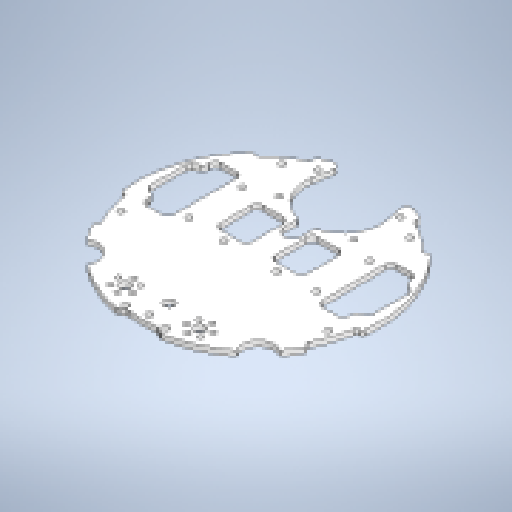
# Autodesk Inventor part: Top Plate
Saved by Autodesk Inventor 2023.2 (Build 272271000, 271)
## iProperties
Created: 2022-12-28
Part Number: Top Plate
Material: UHMW, White
Document SubType Name: Modeling
Designer: Nathan Cai
Mass: 29.6891 g
Surface Area: 260.075 cm^2
Volume: 31.5842 cm^3
Density: 0.94 g/cm^3
Appearance: Smooth - White
Author: Nathan Cai
Autodesk Inventor part; units mm, degrees
ref_plane "YZ Plane" through (0, 0, 0) normal (1, 0, 0) x (0, 1, 0)
ref_plane "XZ Plane" through (0, 0, 0) normal (0, 1, 0) x (-1, 0, 0)
ref_plane "XY Plane" through (0, 0, 0) normal (0, 0, 1) x (1, 0, 0)
sketch "Sketch1" plane through (0, 0, 0) normal (0, 1, 0) x (-1, 0, 0)
  circle A0 centre (0, 0) radius 73.025
  line L0 (0, 0) -> (0, -73.025) construction
  line L1 (0, 0) -> (-12.6807, -71.9156)
  line L2 (0, 0) -> (12.6807, -71.9156)
  line L3 (0, 0) -> (52.5298, -50.7274)
  line L4 (0, 0) -> (32.0121, -65.6344)
  line L5 (0, 0) -> (72.3143, -10.1631)
  line L6 (0, 0) -> (64.4772, -34.2832)
  line L7 (0, 0) -> (64.4772, 34.2832)
  line L8 (0, 0) -> (72.3143, 10.1631)
  line L9 (0, 0) -> (32.0121, 65.6344)
  line L10 (0, 0) -> (52.5298, 50.7274)
  circle A1 centre (0, 0) radius 69.85
  line L11 (0, 0) -> (-12.6807, 71.9156)
  line L12 (0, 0) -> (12.6807, 71.9156)
  line L13 (0, 0) -> (-52.5298, 50.7274)
  line L14 (0, 0) -> (-32.0121, 65.6344)
  line L15 (0, 0) -> (-72.3143, 10.1631)
  line L16 (0, 0) -> (-64.4772, 34.2832)
  line L17 (0, 0) -> (-64.4772, -34.2832)
  line L18 (0, 0) -> (-72.3143, -10.1631)
  line L19 (0, 0) -> (-32.0121, -65.6344)
  line L20 (0, 0) -> (-52.5298, -50.7274)
  point P0 (30.6202, -62.7808)
  point P1 (50.2459, -48.5219)
  point P2 (52.5298, -50.7274)
  point P3 (64.4772, -34.2832)
  point P4 (61.6739, -32.7926)
  point P5 (69.1702, -9.7212)
  point P6 (72.3143, -10.1631)
  point P7 (72.3143, 10.1631)
  point P8 (69.1702, 9.7212)
  point P9 (61.6739, 32.7926)
  point P10 (52.5298, 50.7274)
  point P11 (50.2459, 48.5219)
  point P12 (30.6202, 62.7808)
  point P13 (-12.1293, -68.7888)
  point P14 (12.1293, -68.7888)
  point P15 (12.6807, -71.9156)
  point P16 (32.0121, -65.6344)
  point P17 (12.1293, 68.7888)
  point P18 (-12.1293, 68.7888)
  point P19 (-12.6807, 71.9156)
  point P20 (-64.4772, 34.2832)
  point P21 (-61.6739, 32.7926)
  point P22 (-69.1702, 9.7212)
  point P23 (-52.5298, -50.7274)
  point P24 (-50.2459, -48.5219)
  point P25 (-30.6202, -62.7808)
  dimension "d0" = 146.05
  dimension "d1" = 10
  dimension "d4" = 360
  dimension "d160" = 139.7
  constraints: 42 end point, 4 coincident, 2 centre point, 2 point on circle, 1 symmetric about line, 1 vertical, 49 other
  measures "d0" diameter of A0
  measures "d1" angle of L0 L1
  measures "d160" diameter of A1
extrude "Extrusion1" add sketch "Sketch1" along normal blind 3.175 contours A0 L5 A1 L8 | A0 L6 A1 L5 | L7 A1 L10 A0 | A1 L5 L8 | L8 L7 A1 | A0 L3 A1 L6 | A1 L6 L5 | L10 A1 L9 A0 | L7 L10 A1 | L2 A1 L1 | L4 A1 L2 | L6 A1 L3 | L3 A1 L4 | L12 A1 L9 | L9 A1 L10 | L14 A1 L11 | L11 A1 L12 | L16 A1 L13 | L13 A1 L14 | L18 A1 L15 | L15 A1 L16 | L20 A1 L17 | L17 A1 L18 | L1 A1 L19 | L19 A1 L20 | L9 A1 L12 A0 | A1 L2 A0 L1 | L1 A0 L19 A1 | A1 L4 A0 L2 | A1 L14 A0 L11 | L13 A0 L14 A1 | A1 L16 A0 L13 | A1 L18 A0 L15 | L17 A0 L18 A1 | A1 L20 A0 L17
sketch "Sketch4" plane through (0, 3.175, 0) normal (0, 1, 0) x (1, 0, 0)
  line L0 (0, 0) -> (0, 66.675) construction
  line L1 (-44.45, 26.9875) -> (44.45, 26.9875) construction
  line L2 (44.45, 26.9875) -> (44.45, -1.5875)
  line L3 (44.45, -1.5875) -> (-44.45, -1.5875) construction
  line L4 (-44.45, -1.5875) -> (-44.45, 26.9875)
  line L5 (-44.45, 26.9875) -> (44.45, -1.5875) construction
  line L6 (44.45, 26.9875) -> (-44.45, -1.5875) construction
  line L7 (-44.45, 12.7) -> (44.45, 12.7) construction
  line L8 (-66.675, 34.925) -> (-44.45, 34.925)
  line L9 (-44.45, 34.925) -> (-44.45, -9.525)
  line L10 (-44.45, -9.525) -> (-66.675, -9.525)
  line L11 (-66.675, -9.525) -> (-66.675, 34.925)
  line L12 (-66.675, 34.925) -> (-44.45, -9.525) construction
  line L13 (-44.45, 34.925) -> (-66.675, -9.525) construction
  line L14 (44.45, -1.5875) -> (44.45, 26.9875)
  line L15 (66.675, 34.925) -> (44.45, 34.925)
  line L16 (44.45, 34.925) -> (44.45, -9.525)
  line L17 (44.45, -9.525) -> (66.675, -9.525)
  line L18 (66.675, -9.525) -> (66.675, 34.925)
  line L19 (66.675, 34.925) -> (44.45, -9.525) construction
  line L20 (44.45, 34.925) -> (66.675, -9.525) construction
  line L21 (38.1, 12.7) -> (38.1, 28.575) construction
  circle A0 centre (38.1, 28.575) radius 1.7526
  circle A1 centre (38.1, -3.175) radius 1.7526
  circle A2 centre (-38.1, 28.575) radius 1.7526
  circle A3 centre (-38.1, -3.175) radius 1.7526
  line L22 (-66.675, 34.925) -> (-60.325, 34.925)
  line L23 (-60.325, 34.925) -> (-60.325, 28.575)
  line L24 (-60.325, 28.575) -> (-66.675, 28.575) construction
  line L25 (-66.675, 28.575) -> (-66.675, 34.925)
  line L26 (-60.325, 28.575) -> (-66.675, 24.9088)
  line L27 (-60.325, -9.525) -> (-60.325, -3.175)
  line L28 (-60.325, -3.175) -> (-66.675, 0.4912)
  line L29 (60.325, 34.925) -> (60.325, 28.575)
  line L30 (60.325, 28.575) -> (66.675, 24.9088)
  line L31 (60.325, -9.525) -> (60.325, -3.175)
  line L32 (60.325, -3.175) -> (66.675, 0.4912)
  line L33 (-38.1, -3.175) -> (38.1, -3.175) construction
  circle A4 centre (-15.875, -4.7625) radius 1.7526
  circle A5 centre (15.875, -4.7625) radius 1.7526
  line L34 (-26.0625, 25.4) -> (-7.0125, 25.4)
  line L35 (-7.0125, 25.4) -> (-7.0125, 0)
  line L36 (-7.0125, 0) -> (-26.0625, 0)
  line L37 (-26.0625, 0) -> (-26.0625, 25.4)
  line L38 (-26.0625, 25.4) -> (-7.0125, 0) construction
  line L39 (-7.0125, 25.4) -> (-26.0625, 0) construction
  line L40 (26.0625, 25.4) -> (7.0125, 25.4)
  line L41 (7.0125, 25.4) -> (7.0125, 0)
  line L42 (7.0125, 0) -> (26.0625, 0)
  line L43 (26.0625, 0) -> (26.0625, 25.4)
  line L44 (26.0625, 25.4) -> (7.0125, 0) construction
  line L45 (7.0125, 25.4) -> (26.0625, 0) construction
  circle A6 centre (22.225, -57.15) radius 3.175
  line L46 (22.225, -57.15) -> (28.2642, -55.1877) construction
  circle A7 centre (28.2642, -55.1877) radius 1.5875
  line L47 (22.225, -57.15) -> (22.225, -53.975) construction
  circle A8 centre (26.944, -61.399) radius 1.5875
  circle A9 centre (20.9048, -63.3612) radius 1.5875
  circle A10 centre (16.1858, -59.1123) radius 1.5875
  circle A11 centre (17.506, -52.901) radius 1.5875
  circle A12 centre (23.5452, -50.9388) radius 1.5875
  circle A13 centre (-22.225, -57.15) radius 3.175
  line L48 (-22.225, -57.15) -> (-28.2642, -55.1877) construction
  circle A14 centre (-28.2642, -55.1877) radius 1.5875
  line L49 (-22.225, -57.15) -> (-22.225, -53.975) construction
  circle A15 centre (-26.944, -61.399) radius 1.5875
  circle A16 centre (-20.9048, -63.3612) radius 1.5875
  circle A17 centre (-16.1858, -59.1123) radius 1.5875
  circle A18 centre (-17.506, -52.901) radius 1.5875
  circle A19 centre (-23.5452, -50.9388) radius 1.5875
  point P0 (0, 12.7)
  point P1 (-55.5625, 12.7)
  point P2 (55.5625, 12.7)
  point P3 (44.45, -1.5875)
  point P4 (0, 12.7)
  point P5 (-66.675, 0.4912)
  point P6 (-60.325, -9.525)
  point P7 (-60.325, 34.925)
  point P8 (60.325, -9.525)
  point P9 (66.675, 0.4912)
  point P10 (60.325, 34.925)
  point P11 (-16.5375, 12.7)
  point P12 (16.5375, 12.7)
  dimension "d108" = 6.35
  dimension "d30" = 88.9
  dimension "d31" = 28.575
  dimension "d34" = 22.225
  dimension "d35" = 44.45
  dimension "d52" = 6.35
  dimension "d53" = 15.875
  dimension "d54" = 3.5052
  dimension "d63" = 12.7
  dimension "d64" = 6.35
  dimension "d65" = 6.35
  dimension "d66" = 30
  dimension "d78" = 3.5052
  dimension "d79" = 15.875
  dimension "d80" = 17.4625
  dimension "d104" = 19.05
  dimension "d105" = 25.4
  dimension "d107" = 18.3875
  dimension "d109" = 22.225
  dimension "d110" = 69.85
  dimension "d111" = 6.35
  dimension "d112" = 3.175
  dimension "d113" = 72
  dimension "d116" = 360
  constraints: 100 end point, 32 symmetric about line, 18 centre point, 11 midpoint, 8 parallel, 5 horizontal, 5 point on line, 4 perpendicular, 4 vertical, 3 coincident, 2 vertical alignment, 27 other
  measures "d30" distance of L2.end L3.end
  measures "d31" distance between parallel lines of L3 L1
  measures "d34" distance of L9.end L10.end
  measures "d35" distance of L8.end L9.end
  measures "d52" distance between parallel lines of L16 L21
  measures "d53" distance from line of L7 L21.end
  measures "d54" diameter of A0
  measures "d63" distance of point (0, 12.7) L0.start
  measures "d64" distance of L23.end L24.end
  measures "d65" distance of L22.end L23.end
  measures "d66" angle of L24 L26
  measures "d78" diameter of A4
  measures "d79" distance from line of L0 A4.centre
  measures "d80" distance from line of L7 A4.centre
  measures "d104" distance of L35.end L36.end
  measures "d105" distance of L34.end L35.end
  measures "d107" distance between parallel lines of L4 L37
  measures "d109" horizontal distance of point (0, 12.7) L46.start
  measures "d110" vertical distance of L46.start point (0, 12.7)
  measures "d111" distance of L46.start L46.end
  measures "d112" diameter of A7
  measures "d113" angle of L47 L46
extrude "Extrusion2" cut sketch "Sketch4" against normal through all contours L16 L15 L29 L30 L18 L32 L31 L17 L2 | L9 L10 L27 L28 L11 L26 L23 L8 L4 | A0 | A1 | A2 | A3 | A4 | A5 | L34 L35 L36 L37 | L43 L42 L41 L40 | A6 | A7 | A8 | A9 | A10 | A11 | A12 | A13 | A14 | A15 | A16 | A17 | A18 | A19
fillet "Fillet2" radius 3.175 24 edges at (-44.45, 1.5875, -34.925) (-44.45, 1.5875, 9.525) (44.45, 1.5875, 9.525) (44.45, 1.5875, -34.925) (60.325, 1.5875, -28.575) (66.675, 1.5875, -24.9088) (66.675, 1.5875, -0.4912) (60.325, 1.5875, 3.175) (-60.325, 1.5875, -28.575) (-66.675, 1.5875, -24.9088) (-66.675, 1.5875, -0.4912) (-60.325, 1.5875, 3.175) (60.325, 1.5875, -34.925) (60.325, 1.5875, 9.525) (-60.325, 1.5875, 9.525) (-60.325, 1.5875, -34.925) (-26.0625, 1.5875, -25.4) (-7.0125, 1.5875, -25.4) (-7.0125, 1.5875, 0) (-26.0625, 1.5875, 0) (7.0125, 1.5875, -25.4) (26.0625, 1.5875, -25.4) (26.0625, 1.5875, 0) (7.0125, 1.5875, 0)
sketch "Sketch5" plane through (0, 3.175, 0) normal (0, 1, 0) x (1, 0, 0)
  line L0 (0, 0) -> (0, 66.675) construction
  circle A0 centre (0, 50.8) radius 22.225
  arc A1 (32.0121, 65.6344) -> (-32.0121, 65.6344) centre (0, 0) ccw projected
  circle A2 centre (0, 50.8) radius 17.4625 construction
  circle A3 centre (-24.6063, 60.325) radius 1.7526
  circle A4 centre (-24.6063, 60.325) radius 3.175 construction
  circle A5 centre (-22.225, 34.925) radius 3.175 construction
  circle A6 centre (-22.225, 34.925) radius 1.7526
  circle A7 centre (24.6063, 60.325) radius 1.7526
  circle A8 centre (24.6063, 60.325) radius 3.175 construction
  circle A9 centre (22.225, 34.925) radius 3.175 construction
  circle A10 centre (22.225, 34.925) radius 1.7526
  arc A11 (32.0121, 65.6344) -> (-32.0121, 65.6344) centre (0, 0) ccw projected
  line L1 (-19.05, 70.4964) -> (-21.8767, 54.7195)
  line L2 (19.05, 70.4964) -> (21.8767, 54.7195)
  circle A12 centre (0, 28.575) radius 4.7625
  line L3 (0, 36.5125) -> (0, 20.6375) construction
  line L4 (-4.7625, 36.5125) -> (-4.7625, 20.6375)
  line L5 (4.7625, 20.6375) -> (4.7625, 36.5125)
  arc A13 (4.7625, 36.5125) -> (-4.7625, 36.5125) centre (0, 36.5125) ccw
  arc A14 (-4.7625, 20.6375) -> (4.7625, 20.6375) centre (0, 20.6375) ccw
  point P0 (-30.5456, -66.3296)
  point P1 (12.6807, -71.9156)
  point P2 (64.4772, -34.2832)
  point P3 (-72.5223, -8.5536)
  point P4 (-19.05, 70.4964)
  point P5 (0, 73.025)
  point P6 (21.8767, 54.7195)
  point P7 (19.05, 70.4964)
  point P8 (-4.7351, 29.0853)
  point P9 (4.7351, 29.0853)
  point P10 (0, 15.875)
  point P11 (4.7625, 28.575)
  point P12 (-4.7625, 28.575)
  dimension "d39" = 34.925
  dimension "d40" = 44.45
  dimension "d41" = 3.5052
  dimension "d42" = 6.35
  dimension "d43" = 9.525
  dimension "d44" = 24.6062
  dimension "d45" = 6.35
  dimension "d46" = 3.5052
  dimension "d47" = 15.875
  dimension "d48" = 22.225
  dimension "d74" = 19.05
  dimension "d102" = 9.525
  dimension "d103" = 12.7
  constraints: 14 end point, 13 centre point, 8 point on circle, 7 tangent, 6 symmetric about line, 5 coincident, 3 point on line, 1 midpoint, 1 parallel, 1 vertical, 4 other
  measures "d39" diameter of A2
  measures "d40" diameter of A0
  measures "d41" diameter of A3
  measures "d42" diameter of A4
  measures "d43" vertical distance of A0.centre A3.centre
  measures "d44" horizontal distance of A0.centre A3.centre
  measures "d45" diameter of A5
  measures "d46" diameter of A6
  measures "d47" vertical distance of A0.centre A6.centre
  measures "d48" horizontal distance of A0.centre A6.centre
  measures "d74" distance from line of L0 L1.start
  measures "d102" diameter of A12
  measures "d103" distance of point (0, 15.875) A12.centre
extrude "Extrusion3" cut sketch "Sketch5" against normal blind 25.4 contours A0 L5 A13 L4 | A0 A1 L2 | A0 A12 L4 A13 L5 | A0 L1 A1 | A12 A0 | A0 A12 | L5 A14 L4 A12 | A3 | A6 | A7 | A10
sketch "Sketch6" plane through (0, 0, 0) normal (0, -1, 0) x (1, 0, 0)
  point P0 (11.8537, 67.2254)
  point P1 (-11.8537, 67.2254)
hole "Hole3" at (11.8537, 0, 67.2254) at (-11.8537, 0, 67.2254) direction (0, 1, 0) diameter 3.5052 end through all
sketch "Sketch7" plane through (0, 3.175, 0) normal (0, 1, 0) x (1, 0, 0)
  arc A0 (12.158, -68.9514) -> (11.3889, -68.9153) centre (11.8537, -67.2254) ccw projected
  circle A1 centre (11.8537, -67.2254) radius 3.302
  arc A2 (-11.3889, -68.9153) -> (-12.158, -68.9514) centre (-11.8537, -67.2254) ccw projected
  circle A3 centre (-11.8537, -67.2254) radius 3.302
  circle A4 centre (11.8537, -67.2254) radius 1.7526
  circle A5 centre (-11.8537, -67.2254) radius 1.7526
  point P0 (0, 0)
  point P1 (12.158, -68.9514)
  point P2 (11.3889, -68.9153)
  dimension "d67" = 6.604
  dimension "d68" = 6.604
  constraints: 4 coincident, 3 centre point, 1 concentric, 3 other
  measures "d67" diameter of A1
  measures "d68" diameter of A3
extrude "Extrusion4" add sketch "Sketch7" against normal up to surface (3.175 mm away)
fillet "Fillet4" radius 1.5875 24 edges at (-12.6807, 1.5875, 71.9156) (-12.427, 1.5875, 70.4773) (-9.235, 1.5875, 69.2368) (12.6807, 1.5875, 71.9156) (12.427, 1.5875, 70.4773) (9.235, 1.5875, 69.2368) (69.1702, 1.5875, 9.7212) (72.3143, 1.5875, 10.1631) (64.4772, 1.5875, 34.2832) (61.6739, 1.5875, 32.7926) (30.6202, 1.5875, -62.7808) (32.0121, 1.5875, -65.6344) (52.5298, 1.5875, -50.7274) (50.2459, 1.5875, -48.5219) (-32.0121, 1.5875, -65.6344) (-30.6202, 1.5875, -62.7808) (-52.5298, 1.5875, -50.7274) (-50.2459, 1.5875, -48.5219) (-72.3143, 1.5875, 10.1631) (-69.1702, 1.5875, 9.7212) (-61.6739, 1.5875, 32.7926) (-64.4772, 1.5875, 34.2832) (-4.7351, 1.5875, -29.0853) (4.7351, 1.5875, -29.0853)
fillet "Fillet5" radius 3.175 2 edges at (19.05, 1.5875, -70.4964) (-19.05, 1.5875, -70.4964)
thicken "Thicken1" operation cut thickness 0.25 both sides no extend neighbours no toward (-0.8477101, 0, -0.5304598) faces at (61.904, 2.1167, 38.7368) (63.0601, 1.0583, 33.5296) (63.8199, 1.0583, 34.4266) (13.1942, 1.0583, 71.6582) (62.9587, 1.0583, 33.4709) (12.2225, 1.0583, 70.9396) (66.7871, 2.1167, 20.4576) (9.8443, 2.1167, 69.8457) (70.7248, 1.0583, 9.9397) (69.8129, 1.0583, 10.0825) (8.7126, 2.1167, 69.3268) (70.965, 1.0583, 9.9551) (6.579, 2.1167, 69.5395) (62.1056, 2.1167, -38.4128) (-8.7126, 2.1167, 69.3268) (51.3752, 1.0583, -49.6125) (52.5834, 1.0583, -50.0545) (-9.8443, 1.0583, 69.8457) (50.9955, 1.0583, -49.3411) (-11.7264, 1.0583, 70.5997) (40.0946, 2.1167, -57.1965) (-12.915, 1.0583, 71.5521) (31.3084, 1.0583, -64.1918) (31.1624, 1.0583, -63.2804) (-45.5793, 2.1167, 57.0541) (31.3571, 1.0583, -64.302) (-63.06, 1.0583, 33.5296) (-63.6672, 1.0583, 34.1) (24.8679, 2.1167, -68.6603) (-62.2411, 1.0583, 31.857) (-63.4147, 2.1167, 29.2848) (-70.7249, 1.0583, 9.9397) (-70.2583, 1.0583, 9.9434) (-72.3414, 1.0583, 9.1242) (-72.823, 2.1167, -5.4282) (-51.3752, 1.0583, -49.6124) (-51.8764, 1.0583, -49.9396) (-49.8575, 1.0583, -49.222) (-42.0072, 2.1167, -55.807) (-31.3084, 1.0583, -64.1918) (-31.8083, 1.0583, -62.207) (-31.1844, 1.0583, -65.7948) (-29.847, 2.1167, -66.6469) (19.9211, 2.1167, -65.8489) (21.2411, 2.1167, -58.2668) (13.984, 1.0583, -33.5258) (5.1613, 1.0583, -28.9021) (4.7625, 1.0583, -23.0416) (-2.0416, 1.0583, -16.3348) (-4.7625, 2.1167, -25.4457) (-5.0189, 2.1167, -28.7148) (-19.7168, 1.0583, -40.5434) (-20.6056, 2.1167, -61.8142) (-19.9361, 2.1167, -65.6043)
sketch "Sketch11" plane through (0, 3.175, 0) normal (0, 1, 0) x (1, 0, 0)
  line L0 (-26.9875, -14.2875) -> (-7.9375, -14.2875) construction
  line L1 (-26.9875, -16.6688) -> (-7.9375, -16.6688)
  line L2 (-7.9375, -11.9062) -> (-26.9875, -11.9063)
  arc A0 (-26.9875, -11.9063) -> (-26.9875, -16.6688) centre (-26.9875, -14.2875) ccw
  arc A1 (-7.9375, -16.6688) -> (-7.9375, -11.9062) centre (-7.9375, -14.2875) ccw
  line L3 (-17.4625, -14.2875) -> (-17.4625, -39.6875) construction
  line L4 (-23.8125, -26.9875) -> (-11.1125, -26.9875) construction
  line L5 (-23.8125, -29.3688) -> (-11.1125, -29.3687)
  line L6 (-11.1125, -24.6062) -> (-23.8125, -24.6062)
  arc A2 (-23.8125, -24.6062) -> (-23.8125, -29.3688) centre (-23.8125, -26.9875) ccw
  arc A3 (-11.1125, -29.3687) -> (-11.1125, -24.6062) centre (-11.1125, -26.9875) ccw
  line L7 (-30.1625, -39.6875) -> (-4.7625, -39.6875) construction
  line L8 (-30.1625, -42.0688) -> (-4.7625, -42.0688)
  line L9 (-4.7625, -37.3062) -> (-30.1625, -37.3063)
  arc A4 (-30.1625, -37.3063) -> (-30.1625, -42.0688) centre (-30.1625, -39.6875) ccw
  arc A5 (-4.7625, -42.0688) -> (-4.7625, -37.3062) centre (-4.7625, -39.6875) ccw
  circle A6 centre (-11.1125, -33.3375) radius 2.3813
  line L10 (-17.4625, -39.6875) -> (-17.4625, -14.2875) construction
  line L11 (-15.0813, -39.6875) -> (-15.0812, -14.2875)
  line L12 (-19.8438, -14.2875) -> (-19.8438, -39.6875)
  arc A7 (-19.8438, -39.6875) -> (-15.0813, -39.6875) centre (-17.4625, -39.6875) ccw construction
  arc A8 (-15.0812, -14.2875) -> (-19.8438, -14.2875) centre (-17.4625, -14.2875) ccw construction
  line L13 (20.6375, -14.2875) -> (20.6375, -39.6875) construction
  circle A9 centre (14.2875, -14.2875) radius 2.3813 construction
  line L14 (15.875, -20.6375) -> (15.875, -26.9875) construction
  line L15 (13.4938, -20.6375) -> (13.4938, -26.9875)
  line L16 (18.2563, -26.9875) -> (18.2563, -20.6375)
  arc A10 (18.2563, -20.6375) -> (13.4938, -20.6375) centre (15.875, -20.6375) ccw
  arc A11 (13.4938, -26.9875) -> (18.2563, -26.9875) centre (15.875, -26.9875) ccw
  line L17 (15.875, -20.6375) -> (25.4, -20.6375) construction
  line L18 (15.875, -23.0187) -> (25.4, -23.0187)
  line L19 (25.4, -18.2562) -> (15.875, -18.2562)
  arc A12 (15.875, -18.2562) -> (15.875, -23.0187) centre (15.875, -20.6375) ccw
  arc A13 (25.4, -23.0187) -> (25.4, -18.2562) centre (25.4, -20.6375) ccw
  line L20 (15.875, -26.9875) -> (25.4, -26.9875) construction
  line L21 (15.875, -24.6062) -> (25.4, -24.6062)
  line L22 (25.4, -29.3687) -> (15.875, -29.3687)
  arc A14 (15.875, -24.6062) -> (15.875, -29.3687) centre (15.875, -26.9875) ccw
  arc A15 (25.4, -29.3687) -> (25.4, -24.6062) centre (25.4, -26.9875) ccw
  circle A16 centre (26.9875, -14.2875) radius 2.3813 construction
  line L23 (26.9875, -14.2875) -> (30.1625, -8.7882) construction
  line L24 (29.0497, -15.4781) -> (32.2247, -9.9789)
  line L25 (28.1003, -7.5976) -> (24.9253, -13.0969)
  arc A17 (24.9253, -13.0969) -> (29.0497, -15.4781) centre (26.9875, -14.2875) ccw
  arc A18 (32.2247, -9.9789) -> (28.1003, -7.5976) centre (30.1625, -8.7882) ccw
  line L26 (26.9875, -14.2875) -> (33.3375, -14.2875) construction
  line L27 (14.2875, -14.2875) -> (11.1125, -8.7882) construction
  line L28 (16.3497, -13.0969) -> (13.1747, -7.5976)
  line L29 (9.0503, -9.9789) -> (12.2253, -15.4781)
  arc A19 (12.2253, -15.4781) -> (16.3497, -13.0969) centre (14.2875, -14.2875) ccw
  arc A20 (13.1747, -7.5976) -> (9.0503, -9.9789) centre (11.1125, -8.7882) ccw
  line L30 (14.2875, -14.2875) -> (20.6375, -14.2875) construction
  line L31 (11.1125, -33.3375) -> (11.1125, -39.6875) construction
  line L32 (8.7313, -33.3375) -> (8.7313, -39.6875)
  line L33 (13.4938, -39.6875) -> (13.4938, -33.3375)
  arc A21 (13.4938, -33.3375) -> (8.7313, -33.3375) centre (11.1125, -33.3375) ccw
  arc A22 (8.7313, -39.6875) -> (13.4938, -39.6875) centre (11.1125, -39.6875) ccw
  line L34 (17.4625, -33.3375) -> (17.4625, -39.6875) construction
  line L35 (15.0813, -33.3375) -> (15.0813, -39.6875)
  line L36 (19.8438, -39.6875) -> (19.8438, -33.3375)
  arc A23 (19.8438, -33.3375) -> (15.0813, -33.3375) centre (17.4625, -33.3375) ccw
  arc A24 (15.0813, -39.6875) -> (19.8438, -39.6875) centre (17.4625, -39.6875) ccw
  line L37 (17.4625, -39.6875) -> (30.1625, -39.6875) construction
  line L38 (17.4625, -37.3062) -> (30.1625, -37.3062)
  line L39 (30.1625, -42.0688) -> (17.4625, -42.0688)
  arc A25 (17.4625, -37.3062) -> (17.4625, -42.0688) centre (17.4625, -39.6875) ccw
  arc A26 (30.1625, -42.0688) -> (30.1625, -37.3062) centre (30.1625, -39.6875) ccw
  circle A27 centre (23.8125, -33.3375) radius 2.3813
  circle A28 centre (30.1625, -33.3375) radius 2.3813
  line L40 (17.4625, -33.3375) -> (30.1625, -33.3375) construction
  line L41 (30.1625, -33.3375) -> (30.1625, -39.6875) construction
  arc A29 (53.6121, -36.9069) -> (36.9069, -53.6121) centre (52.759, -52.759) ccw construction
  arc A30 (53.7828, -33.7365) -> (33.7365, -53.7828) centre (52.759, -52.759) ccw
  arc A31 (53.4415, -40.0774) -> (40.0774, -53.4415) centre (52.759, -52.759) ccw
  arc A32 (53.4415, -40.0774) -> (53.7828, -33.7365) centre (53.6121, -36.9069) ccw
  arc A33 (33.7365, -53.7828) -> (40.0774, -53.4415) centre (36.9069, -53.6121) ccw
  circle A34 centre (0, 0) radius 65.0875 construction
  line L42 (0, 0) -> (41.5337, -41.5337) construction
  circle A35 centre (0, -64.525) radius 3 projected
  line L43 (0, 0) -> (0, -64.525) construction
  circle A36 centre (52.759, -52.759) radius 9.525
  arc A37 (-36.9069, -53.6121) -> (-53.6121, -36.9069) centre (-52.759, -52.759) ccw construction
  arc A38 (-33.7365, -53.7828) -> (-53.7828, -33.7365) centre (-52.759, -52.759) ccw
  arc A39 (-40.0774, -53.4415) -> (-53.4415, -40.0774) centre (-52.759, -52.759) ccw
  arc A40 (-53.7828, -33.7365) -> (-53.4415, -40.0774) centre (-53.6121, -36.9069) ccw
  arc A41 (-40.0774, -53.4415) -> (-33.7365, -53.7828) centre (-36.9069, -53.6121) ccw
  circle A42 centre (-52.759, -52.759) radius 9.525
  point P0 (-17.4625, -26.9875)
  point P1 (15.875, -23.8125)
  point P2 (20.6375, -20.6375)
  point P3 (20.6375, -26.9875)
  point P4 (20.6375, -26.9875)
  point P5 (28.575, -11.5379)
  point P6 (12.7, -11.5379)
  point P7 (11.1125, -36.5125)
  point P8 (17.4625, -36.5125)
  point P9 (23.8125, -39.6875)
  point P10 (-19.8438, -29.3688)
  point P11 (-19.8438, -37.3062)
  point P12 (-15.0813, -37.3062)
  point P13 (-15.0813, -29.3687)
  point P14 (-15.0812, -24.6062)
  point P15 (-15.0812, -16.6688)
  point P16 (-19.8438, -16.6688)
  point P17 (-19.8438, -24.6062)
  point P18 (15.875, -18.2562)
  point P19 (18.2563, -24.6062)
  point P20 (18.2563, -23.0187)
  point P21 (19.8438, -37.3062)
  dimension "d118" = 9.525
  dimension "d119" = 4.7625
  dimension "d120" = 25.4
  dimension "d121" = 2.3813
  dimension "d122" = 6.35
  dimension "d123" = 2.3813
  dimension "d124" = 12.7
  dimension "d125" = 4.7625
  dimension "d126" = 6.35
  dimension "d127" = 6.35
  dimension "d128" = 26.9875
  dimension "d129" = 17.4625
  dimension "d130" = 2.3813
  dimension "d131" = 20.6375
  dimension "d132" = 4.7625
  dimension "d133" = 3.175
  dimension "d134" = 4.7625
  dimension "d135" = 4.7625
  dimension "d136" = 2.3813
  dimension "d137" = 26.9875
  dimension "d138" = 6.35
  dimension "d139" = 6.35
  dimension "d140" = 6.35
  dimension "d141" = 60
  dimension "d142" = 6.35
  dimension "d143" = 120
  dimension "d144" = 2.3813
  dimension "d145" = 2.3813
  dimension "d146" = 3.175
  dimension "d147" = 25.4
  dimension "d148" = 6.35
  dimension "d149" = 6.35
  dimension "d150" = 4.7625
  dimension "d151" = 4.7625
  dimension "d152" = 6.35
  dimension "d155" = 6.35
  dimension "d156" = 130.175
  dimension "d157" = 15.875
  dimension "d158" = 45
  dimension "d159" = 19.05
  constraints: 112 end point, 74 point on circle, 53 tangent, 42 centre point, 17 equal length, 16 midpoint, 8 symmetric about line, 6 horizontal, 6 point on line, 5 vertical, 4 coincident, 3 perpendicular, 2 concentric, 6 other
  measures "d118" distance of L3.start L0.end
  measures "d119" diameter of A1
  measures "d120" distance of L3.start L3.end
  measures "d121" radius of A3
  measures "d122" distance of L4.end point (-17.463, -26.988)
  measures "d123" radius of A5
  measures "d124" distance of L7.end L3.end
  measures "d125" diameter of A6
  measures "d126" distance from line of L3 A6.centre
  measures "d127" distance from line of L4 A6.centre
  measures "d128" vertical distance of point (0, 0) point (-17.463, -26.988)
  measures "d129" horizontal distance of point (0, 0) point (-17.463, -26.988)
  measures "d130" radius of A8
  measures "d131" horizontal distance of point (20.638, -26.988) point (0, 0)
  measures "d132" diameter of A9
  measures "d133" distance of point (15.875, -23.812) L14.end
  measures "d134" diameter of A16
  measures "d135" distance between parallel lines of L13 L14
  measures "d136" radius of A13
  measures "d137" vertical distance of point (0, 0) point (20.638, -26.988)
  measures "d138" distance from line of L13 L27.start
  measures "d139" distance from line of L13 L23.start
  measures "d140" distance of L23.start L23.end
  measures "d141" angle of L26 L23
  measures "d142" distance of L27.start L27.end
  measures "d143" angle of L30 L27
  measures "d144" radius of A26
  measures "d145" radius of A21
  measures "d146" distance between parallel lines of L34 L13
  measures "d147" distance of L13.start L13.end
  measures "d148" distance of L34.end L34.start
  measures "d149" distance of L37.end point (23.813, -39.688)
  measures "d150" diameter of A27
  measures "d151" diameter of A28
  measures "d152" distance between parallel lines of L34 L31
  measures "d155" diameter of A33
  measures "d156" diameter of A34
  measures "d157" radius of A29
  measures "d158" angle of L43 L42
  measures "d159" diameter of A36
extrude "Extrusion5" cut sketch "Sketch11" against normal through all contours A36 | A42
sketch "Sketch12" plane through (0, 3.175, 0) normal (0, 1, 0) x (1, 0, 0)
  point P0 (0, -65.0875)
  point P1 (11.8537, -67.2254)
  point P2 (-11.8537, -67.2254)
  point P3 (-61.9019, -20.1131)
  point P4 (15.875, -4.7625)
  point P5 (-15.875, -4.7625)
  point P6 (61.9019, -20.1131)
  point P7 (-38.2575, 52.6569)
  point P8 (38.2575, 52.6569)
  point P9 (38.1, -3.175)
  point P10 (38.1, 28.575)
  point P11 (-38.1, 28.575)
  point P12 (-38.1, -3.175)
hole "Hole7" at (0, 3.175, 65.0875) at (11.8537, 3.175, 67.2254) at (-11.8537, 3.175, 67.2254) at (-61.9019, 3.175, 20.1131) at (15.875, 3.175, 4.7625) at (-15.875, 3.175, 4.7625) at (61.9019, 3.175, 20.1131) at (-38.2575, 3.175, -52.6569) at (38.2575, 3.175, -52.6569) at (38.1, 3.175, 3.175) at (38.1, 3.175, -28.575) at (-38.1, 3.175, -28.575) at (-38.1, 3.175, 3.175) direction (0, -1, 0) diameter 3.7973 end through all
sketch "Sketch13" plane through (0, 3.175, 0) normal (0, 1, 0) x (1, 0, 0)
  circle A0 centre (0, -65.0875) radius 1.8986 projected
  circle A1 centre (0, -65.0875) radius 6.35 construction
  line L0 (0, 0) -> (0, -65.0875) construction
  circle A2 centre (0, -53.1812) radius 5.5563 construction
  circle A3 centre (0, -53.1812) radius 3.175
  dimension "d168" = 12.7
  dimension "d169" = 11.1125
  dimension "d170" = 6.35
  constraints: 3 centre point, 2 coincident, 2 end point, 1 point on line, 1 tangent, 1 vertical
  measures "d168" diameter of A1
  measures "d169" diameter of A2
  measures "d170" diameter of A3
extrude "Extrusion6" cut sketch "Sketch13" against normal through all contours A3
equation "\"d45\" = d42"
equation "\"d46\" = d41"
body "Solid1"
